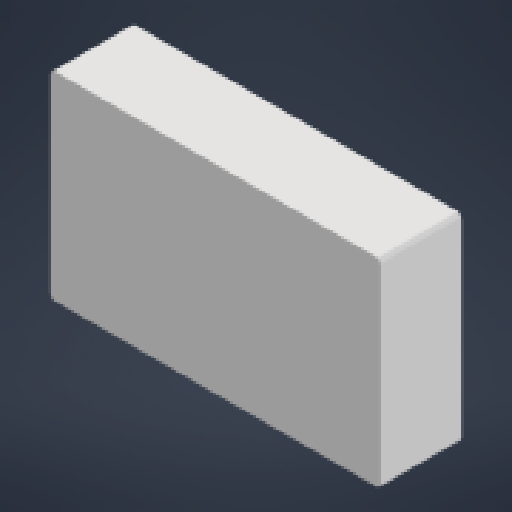
# Autodesk Inventor part: case
Saved by Autodesk Inventor 2023.2 (Build 272271000, 271)
## iProperties
Created: 2023-01-24
Part Number: case
Material: Generic
Document SubType Name: Modeling
Designer: adnew
Density: 1 g/cm^3
Appearance: Default
Author: adnew
Autodesk Inventor part; units mm, degrees
ref_plane "YZ Plane" through (0, 0, 0) normal (1, 0, 0) x (0, 1, 0)
ref_plane "XZ Plane" through (0, 0, 0) normal (0, 1, 0) x (-1, 0, 0)
ref_plane "XY Plane" through (0, 0, 0) normal (0, 0, 1) x (1, 0, 0)
sketch "Sketch1" plane through (0, 0, 0) normal (0, 0, 1) x (1, 0, 0)
  line L0 (-36, 20.9) -> (-36, -20.9) construction
  line L1 (-36, -20.9) -> (36, -20.9) construction
  line L2 (36, -20.9) -> (36, 20.9) construction
  line L3 (36, 20.9) -> (-36, 20.9) construction
  circle A0 centre (-20, -13.1) radius 1.6 construction
  circle A1 centre (-30.3, -1.8) radius 0.65 construction
  circle A2 centre (27.2, -13.1) radius 1.6 construction
  circle A3 centre (-30.3, 3.2) radius 0.65 construction
  circle A4 centre (-20, 13.1) radius 1.6 construction
  circle A5 centre (27.2, 13.1) radius 1.6 construction
  line L4 (-38, 21.9) -> (-38, -21.9)
  line L5 (-37, -22.9) -> (37, -22.9)
  line L6 (38, -21.9) -> (38, 21.9)
  line L7 (37, 22.9) -> (-37, 22.9)
  arc A6 (-37, 22.9) -> (-38, 21.9) centre (-37, 21.9) ccw
  arc A7 (38, 21.9) -> (37, 22.9) centre (37, 21.9) ccw
  arc A8 (37, -22.9) -> (38, -21.9) centre (37, -21.9) ccw
  arc A9 (-38, -21.9) -> (-37, -22.9) centre (-37, -21.9) ccw
  line L8 (-38, -9.1) -> (-20, -9.1)
  line L9 (-16, -13.1) -> (-16, -22.9)
  arc A10 (-16, -13.1) -> (-20, -9.1) centre (-20, -13.1) ccw
  line L10 (-38, 9.1) -> (-20, 9.1)
  line L11 (-16, 13.1) -> (-16, 20.9)
  line L12 (23.2, -22.9) -> (23.2, -13.1)
  line L13 (27.2, -9.1) -> (38, -9.1)
  line L14 (38, 9.1) -> (27.2, 9.1)
  line L15 (23.2, 13.1) -> (23.2, 22.9)
  arc A11 (-20, 9.1) -> (-16, 13.1) centre (-20, 13.1) ccw
  arc A12 (27.2, -9.1) -> (23.2, -13.1) centre (27.2, -13.1) ccw
  arc A13 (23.2, 13.1) -> (27.2, 9.1) centre (27.2, 13.1) ccw
  line L16 (-16, 20.9) -> (-16, 22.9)
  line L17 (-36, -9.1) -> (-36, 9.1)
  line L18 (-16, 20.9) -> (23.2, 20.9)
  line L19 (36, 9.1) -> (36, -9.1)
  line L20 (23.2, -20.9) -> (-16, -20.9)
  line L21 (34, -18.9) -> (-34, -18.9)
  line L22 (-34, -18.9) -> (-34, 18.9)
  line L23 (-34, 18.9) -> (34, 18.9)
  line L24 (34, 18.9) -> (34, -18.9)
  point P0 (0, 0)
  point P1 (23.2, 9.1)
  point P2 (-16, 18.9)
  point P3 (23.2, 18.9)
  point P4 (34, 9.1)
  point P5 (34, -9.1)
  point P6 (23.2, -18.9)
  point P7 (-16, -18.9)
  point P8 (-34, -9.1)
  point P9 (-34, 9.1)
  dimension "d0" = 2
  dimension "d1" = 1
  dimension "d2" = 4
  dimension "d3" = 4
  dimension "d4" = 4
  dimension "d5" = 4
  dimension "d6" = 2
  constraints: 42 end point, 27 point on line, 16 point on circle, 16 tangent, 8 centre point, 6 perpendicular, 4 coincident, 3 equal radius, 1 horizontal, 1 vertical, 6 other
  measures "d0" distance between parallel lines of L4 L0
  measures "d1" radius of A6
  measures "d2" radius of A10
  measures "d3" radius of A11
  measures "d4" radius of A12
  measures "d5" radius of A13
  measures "d6" distance between parallel lines of L1 L21
extrude "Extrusion1" add sketch "Sketch1" along normal blind 15 contours A6 L7 L16 L11 L23 L22 L10 L4 | L10 L17 L8 L4 | L8 L22 L21 L9 L5 A9 L4 | L10 L22 L8 L17 | L7 L15 L18 L16 | L22 L23 L11 A11 L10 | L7 A7 L6 L14 L24 L23 L15 | L18 L15 L23 L11 | L8 A10 L9 L21 L22 | L9 L20 L12 L5 | L23 L24 L14 A13 L15 | L12 L21 L24 L13 L6 A8 L5 | L9 L21 L12 L20 | L6 L13 L19 L14 | L12 A12 L13 L24 L21 | L19 L13 L24 L14
sketch "Sketch2" plane through (0, 0, 15) normal (0, 0, 1) x (1, 0, 0)
  line L0 (37, 22.9) -> (-37, 22.9) projected
  arc A0 (-37, 22.9) -> (-38, 21.9) centre (-37, 21.9) ccw projected
  line L1 (-38, 21.9) -> (-38, -21.9) projected
  line L2 (-37, -22.9) -> (37, -22.9) projected
  arc A1 (-38, -21.9) -> (-37, -22.9) centre (-37, -21.9) ccw projected
  arc A2 (37, -22.9) -> (38, -21.9) centre (37, -21.9) ccw projected
  line L3 (38, -21.9) -> (38, 21.9) projected
  arc A3 (38, 21.9) -> (37, 22.9) centre (37, 21.9) ccw projected
  point P0 (0, 0)
extrude "Extrusion2" add sketch "Sketch2" along normal blind 2
sketch "Sketch3" plane through (0, 0, 0) normal (0, 0, -1) x (-1, 0, 0)
  arc A0 (-37, 22.9) -> (-38, 21.9) centre (-37, 21.9) ccw projected
  line L0 (-37, 22.9) -> (37, 22.9) projected
  line L1 (-38, -21.9) -> (-38, 21.9) projected
  arc A1 (-38, -21.9) -> (-37, -22.9) centre (-37, -21.9) ccw projected
  line L2 (37, -22.9) -> (-37, -22.9) projected
  arc A2 (37, -22.9) -> (38, -21.9) centre (37, -21.9) ccw projected
  line L3 (38, 21.9) -> (38, -21.9) projected
  arc A3 (38, 21.9) -> (37, 22.9) centre (37, 21.9) ccw projected
  line L4 (-36, 20.9) -> (36, 20.9) projected
  line L5 (-36, -20.9) -> (-36, 20.9) projected
  line L6 (36, -20.9) -> (-36, -20.9) projected
  line L7 (36, 20.9) -> (36, -20.9) projected
  point P0 (0, 0)
extrude "Extrusion3" add sketch "Sketch3" along normal blind 1.5
sketch "Sketch4" plane through (0, 0, 0) normal (0, 0, -1) x (-1, 0, 0)
  circle A0 centre (-27.2, 13.1) radius 2.585
  arc A1 (-27.2, 11.656624) -> (-25.95, 12.378312) centre (-27.2, 13.1) ccw
  arc A2 (-28.45, 12.378312) -> (-27.2, 11.656624) centre (-27.2, 13.1) ccw
  arc A3 (-28.45, 13.821688) -> (-28.45, 12.378312) centre (-27.2, 13.1) ccw
  arc A4 (-27.2, 14.543376) -> (-28.45, 13.821688) centre (-27.2, 13.1) ccw
  arc A5 (-25.95, 13.821688) -> (-27.2, 14.543376) centre (-27.2, 13.1) ccw
  arc A6 (-25.95, 12.378312) -> (-25.95, 13.821688) centre (-27.2, 13.1) ccw
  circle A7 centre (20, 13.1) radius 2.585
  arc A8 (20, 11.656624) -> (21.25, 12.378312) centre (20, 13.1) ccw
  arc A9 (18.75, 12.378312) -> (20, 11.656624) centre (20, 13.1) ccw
  arc A10 (18.75, 13.821688) -> (18.75, 12.378312) centre (20, 13.1) ccw
  arc A11 (20, 14.543376) -> (18.75, 13.821688) centre (20, 13.1) ccw
  arc A12 (21.25, 13.821688) -> (20, 14.543376) centre (20, 13.1) ccw
  arc A13 (21.25, 12.378312) -> (21.25, 13.821688) centre (20, 13.1) ccw
  circle A14 centre (20, -13.1) radius 2.585
  arc A15 (20, -14.543376) -> (21.25, -13.821688) centre (20, -13.1) ccw
  arc A16 (18.75, -13.821688) -> (20, -14.543376) centre (20, -13.1) ccw
  arc A17 (18.75, -12.378312) -> (18.75, -13.821688) centre (20, -13.1) ccw
  arc A18 (20, -11.656624) -> (18.75, -12.378312) centre (20, -13.1) ccw
  arc A19 (21.25, -12.378312) -> (20, -11.656624) centre (20, -13.1) ccw
  arc A20 (21.25, -13.821688) -> (21.25, -12.378312) centre (20, -13.1) ccw
  circle A21 centre (-27.2, -13.1) radius 2.585
  arc A22 (-27.2, -14.543376) -> (-25.95, -13.821688) centre (-27.2, -13.1) ccw
  arc A23 (-28.45, -13.821688) -> (-27.2, -14.543376) centre (-27.2, -13.1) ccw
  arc A24 (-28.45, -12.378312) -> (-28.45, -13.821688) centre (-27.2, -13.1) ccw
  arc A25 (-27.2, -11.656624) -> (-28.45, -12.378312) centre (-27.2, -13.1) ccw
  arc A26 (-25.95, -12.378312) -> (-27.2, -11.656624) centre (-27.2, -13.1) ccw
  arc A27 (-25.95, -13.821688) -> (-25.95, -12.378312) centre (-27.2, -13.1) ccw
  point P0 (0, 0)
hole "Hole1" at (27.2, 13.1, 0) at (-20, 13.1, 0) at (-20, -13.1, 0) at (27.2, -13.1, 0) direction (0, 0, 1) diameter 3 depth 8
sketch "Sketch5" plane through (-38, -21.9, 17) normal (-1, 0, 0) x (0, 0, 1)
  line L0 (-2, 12.8) -> (-2, 31) projected
  line L1 (-17, 12.8) -> (-2, 12.8) projected
  point P0 (-17, 21.9)
  point P1 (-7, 21.9)
  dimension "d20" = 5
  dimension "d21" = 9.1
  measures "d20" distance from line of point (-7, 21.9) L0
  measures "d21" distance from line of point (-7, 21.9) L1
hole "Hole2" at (-38, 0, 10) direction (1, 0, 0) diameter 4.7 depth 8
sketch "Sketch7" plane through (-34, -9.1, 0) normal (1, 0, 0) x (0, 0, -1)
  circle A0 centre (-10, 9.1) radius 2.35 projected
  line L0 (-10, 11.45) -> (-10, 13.1)
  line L1 (-10, 13.1) -> (-15, 13.1)
  line L2 (-15, 13.1) -> (-15, 5.1)
  line L3 (-15, 0) -> (-15, 18.2) projected
  line L4 (-15, 5.1) -> (-10, 5.1)
  line L5 (-10, 5.1) -> (-10, 6.75)
  point P0 (0, 9.1)
  dimension "d29" = 8
  dimension "d30" = 5
  constraints: 10 end point, 4 collinear, 2 perpendicular, 2 point on circle, 1 point on line, 1 vertical
  measures "d29" distance of L1.end L2.end
  measures "d30" distance between parallel lines of L2 L5
extrude "Extrusion4" add sketch "Sketch7" along normal blind 6.35 contours A0 L5 L4 L2 L1 L0
sketch "Sketch8" plane through (-34, -4, 10) normal (0, -1, 0) x (1, 0, 0)
  line L0 (0, 5) -> (6.35, 5) projected
  line L1 (5.35, 5) -> (1.54, 5)
  line L2 (1.54, 5) -> (1.54, 3.095)
  line L3 (1.54, 3.095) -> (5.35, 3.095)
  line L4 (5.35, 3.095) -> (5.35, 5)
  line L5 (6.35, 5) -> (6.35, 0) projected
  point P0 (34, -10)
  point P1 (1.54, 5)
  dimension "d33" = 3.81
  dimension "d34" = 1.905
  dimension "d35" = 1
  constraints: 8 end point, 2 parallel, 1 horizontal, 1 perpendicular, 1 point on line
  measures "d33" distance of L2.end L3.end
  measures "d34" distance between parallel lines of L1 L3
  measures "d35" distance between parallel lines of L4 L5
extrude "Extrusion5" cut sketch "Sketch8" against normal up to surface (8 mm away)
fillet "Fillet1" radius 1 2 edges at (-30.825, 4, 10) (-30.825, -4, 10)
fillet "Fillet2" radius 1 8 edges at (37.7071, -22.6071, 17) (38, 0, 17) (37.7071, 22.6071, 17) (0, 22.9, 17) (-37.7071, 22.6071, 17) (-38, 0, 17) (-37.7071, -22.6071, 17) (0, -22.9, 17)
ref_plane "Work Plane3" through (18.5, 21.9, 17) normal (0, -0.7071068, 0.7071068) x (1, 0, 0)
sketch "Sketch9" plane through (18.5, 21.9, 17) normal (0, -0.7071068, 0.7071068) x (1, 0, 0)
  line L0 (-51.5, -2.77) -> (-47.69, -2.77)
  line L1 (-47.69, -2.77) -> (-47.69, -1.5)
  line L2 (-47.69, -1.5) -> (-51.5, -1.5)
  line L3 (-51.5, -1.5) -> (-51.5, -2.77)
  line L4 (10.69, -2.77) -> (14.5, -2.77)
  line L5 (14.5, -2.77) -> (14.5, -1.5)
  line L6 (14.5, -1.5) -> (10.69, -1.5)
  line L7 (10.69, -1.5) -> (10.69, -2.77)
  line L8 (-56.5, -0.707107) -> (-56.5, -31.678384)
  line L9 (19.5, -31.678384) -> (19.5, -0.707107)
  line L10 (18.5, -30.971277) -> (-55.5, -30.971277)
  line L11 (18.5, 0) -> (18.5, -30.971277)
  line L12 (-55.5, 0) -> (18.5, 0)
  line L13 (-55.5, -30.971277) -> (-55.5, 0)
  point P0 (-18.5, -27.506454)
  dimension "d42" = 3.81
  dimension "d43" = 1.27
  dimension "d44" = 5
  dimension "d45" = 5
  dimension "d46" = 1.5
  constraints: 16 end point, 4 parallel, 2 horizontal, 2 perpendicular, 2 point on line, 1 collinear
  measures "d42" distance of L1.end L2.end
  measures "d43" distance of L4.end L5.end
  measures "d44" distance between parallel lines of L3 L8
  measures "d45" distance between parallel lines of L9 L5
  measures "d46" distance between parallel lines of L2 L12
extrude "Extrusion6" cut sketch "Sketch9" along normal through all both and the other way through all contours L3 L2 L1 L0 | L7 L6 L5 L4
ref_plane "Work Plane4" through (-37, 0, -1.5) normal (0, 1, 0) x (1, 0, 0)
mirror "Mirror1" about plane through (-37, 0, -1.5) normal (0, 1, 0) of "Extrusion6"
fillet "Fillet3" radius 1 8 edges at (-37.7071, -22.6071, -1.5) (-38, 0, -1.5) (-37.7071, 22.6071, -1.5) (0, 22.9, -1.5) (37.7071, 22.6071, -1.5) (38, 0, -1.5) (37.7071, -22.6071, -1.5) (0, -22.9, -1.5)
body "Solid1"
